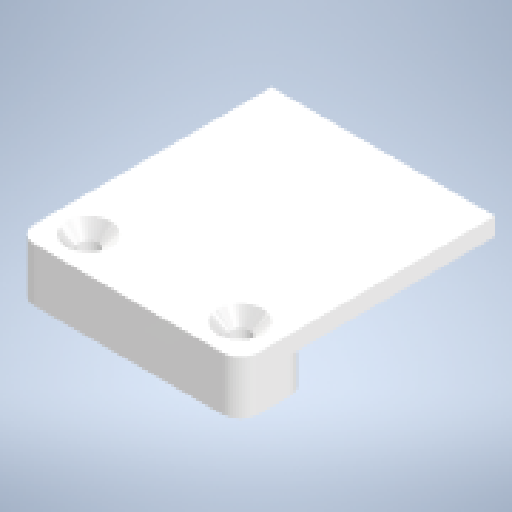
# Autodesk Inventor part: Sliderhalter
Saved by Autodesk Inventor 2025 (Build 290162010, 162A)
## iProperties
Created: 2024-11-26
Part Number: Sliderhalter
Material: PC/ABS-Kunststoff, 3DDruck, PLA
Document SubType Name: Modeling
Designer: Admin
Density: 1.1 g/cm^3
Appearance: Glatt - Weiß(2)
Author: Admin
Autodesk Inventor part; units mm, degrees
ref_plane "YZ Plane" through (0, 0, 0) normal (1, 0, 0) x (0, 1, 0)
ref_plane "XZ Plane" through (0, 0, 0) normal (0, 1, 0) x (-1, 0, 0)
ref_plane "XY Plane" through (0, 0, 0) normal (0, 0, 1) x (1, 0, 0)
sketch "Skizze1" plane through (0, 0, 0) normal (0, 0, 1) x (1, 0, 0)
  line L0 (75.1333, -4.3546) -> (75.1333, -11.8546)
  line L1 (75.1333, -11.8546) -> (50.1333, -11.8546)
  line L2 (50.1333, -11.8546) -> (50.1333, -4.3546)
  line L3 (50.1333, -4.3546) -> (75.1333, -4.3546)
  point P0 (0, 0)
  dimension "d1" = 7.5
  dimension "d2" = 25
  constraints: 8 end point, 2 perpendicular, 1 horizontal, 1 parallel
  measures "d1" distance of L0.end L0.start
  measures "d2" distance of L0.start L2.end
extrude "Extrusion1" add sketch "Skizze1" along normal blind 4
sketch "Skizze2" plane through (0, 0, 4) normal (0, 0, 1) x (1, 0, 0)
  line L0 (75.1333, 16.6454) -> (50.1333, 16.6454)
  line L1 (50.1333, 16.6454) -> (50.1333, -4.3546)
  line L2 (75.1333, -4.3546) -> (75.1333, 16.6454)
  line L3 (50.1333, -11.8546) -> (75.1333, -11.8546) projected
  line L4 (75.1333, -11.8546) -> (75.1333, -4.3546) projected
  line L5 (50.1333, -4.3546) -> (50.1333, -11.8546) projected
  line L6 (50.1333, 16.6454) -> (45.1333, 16.6454)
  line L7 (45.1333, 16.6454) -> (45.1333, 11.6454)
  line L8 (45.1333, 11.6454) -> (50.1333, 11.6454)
  line L9 (50.1333, 11.6454) -> (50.1333, 16.6454)
  line L10 (75.1333, 16.6454) -> (80.1333, 16.6454)
  line L11 (80.1333, 16.6454) -> (80.1333, 11.6454)
  line L12 (80.1333, 11.6454) -> (75.1333, 11.6454)
  line L13 (75.1333, 11.6454) -> (75.1333, 16.6454)
  point P0 (0, 0)
  dimension "d25" = 28.5
  dimension "d28" = 5
  dimension "d29" = 5
  constraints: 22 end point, 4 parallel, 3 perpendicular, 2 collinear, 2 horizontal, 1 point on line, 1 vertical
  measures "d25" distance between parallel lines of L0 L3
  measures "d28" distance of L8.end L7.end
  measures "d29" distance of L7.end L6.end
extrude "Extrusion2" add sketch "Skizze2" along normal blind 3 contours L2 L4 L3 L5 L1 L0
sketch "Skizze3" plane through (0, 0, 7) normal (0, 0, 1) x (1, 0, 0)
  line L0 (50.1333, 16.6454) -> (50.1333, -11.8546) projected
  line L1 (54.1333, -7.8546) -> (50.1333, -7.8546) construction
  line L2 (54.1333, -7.8546) -> (54.1333, -11.8546) construction
  line L3 (71.1333, -7.8546) -> (71.1333, -11.8546) construction
  line L4 (71.1333, -7.8546) -> (75.1333, -7.8546) construction
  line L5 (50.1333, -11.8546) -> (75.1333, -11.8546) construction
  line L6 (75.1333, -11.8546) -> (75.1333, 16.6454) construction
  point P0 (0, 0)
  dimension "d26" = 4
  constraints: 8 end point, 4 point on line, 3 equal length, 2 vertical, 1 horizontal, 1 perpendicular
  measures "d26" distance from line of L0 L1.start
hole "Bohrung1" at (54.1333, -7.8546, 7) at (71.1333, -7.8546, 7) direction (0, 0, -1) diameter 2.2 end through all countersink diameter 5 countersink angle 90
fillet "Rundung1" radius 2 4 edges at (50.1333, -11.8546, 3.5) (75.1333, -11.8546, 3.5) (75.1333, -4.3546, 2) (50.1333, -4.3546, 2)
sketch "Skizze4" plane through (0, 0, 7) normal (0, 0, 1) x (1, 0, 0)
  line L0 (75.1333, -6.3546) -> (75.1333, 16.6454) projected
  line L1 (81.1333, 16.6454) -> (75.1333, 16.6454)
  line L2 (75.1333, 16.6454) -> (75.1333, 11.6454)
  line L3 (75.1333, 11.6454) -> (81.1333, 11.6454)
  line L4 (81.1333, 11.6454) -> (81.1333, 16.6454)
  line L5 (75.1333, 16.6454) -> (50.1333, 16.6454) projected
  line L6 (50.1333, 16.6454) -> (44.1333, 16.6454)
  line L7 (44.1333, 16.6454) -> (44.1333, 11.6454)
  line L8 (44.1333, 11.6454) -> (50.1333, 11.6454)
  line L9 (50.1333, 11.6454) -> (50.1333, 16.6454)
  point P0 (0, 0)
  dimension "d30" = 5
  dimension "d31" = 6
  constraints: 16 end point, 4 parallel, 2 equal length, 2 horizontal, 2 perpendicular, 1 point on line
  measures "d30" distance of L3.end L1.start
  measures "d31" distance of L2.end L3.end
extrude "Extrusion3" add sketch "Skizze4" against normal blind 2
sketch "Skizze5" plane through (0, 0, 7) normal (0, 0, 1) x (1, 0, 0)
  line L0 (44.1333, 11.6454) -> (44.1333, 16.6454) projected
  line L1 (44.1333, 14.1454) -> (46.6333, 14.1454)
  line L2 (78.6333, 14.1454) -> (81.1333, 14.1454)
  line L3 (81.1333, 11.6454) -> (81.1333, 16.6454) projected
  line L4 (44.1333, 11.6454) -> (50.1333, 11.6454) projected
  point P0 (0, 0)
  dimension "d34" = 2.5
  dimension "d42" = 2.5
  dimension "d43" = 2.5
  constraints: 4 end point, 2 horizontal, 2 midpoint, 1 collinear
  measures "d34" distance of L1.start L1.end
  measures "d42" distance between parallel lines of L4 L1
  measures "d43" horizontal distance of L0.end L1.end
hole "Bohrung2" at (78.6333, 14.1454, 7) at (46.6333, 14.1454, 7) direction (0, 0, -1) diameter 2.2 end through all countersink diameter 4.4 countersink angle 90 clearance for "Flachkopfmaschinenschraube" size "M2" standard "ANSI Metrisches M Profil"
